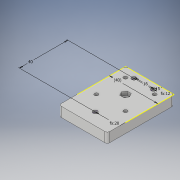
# Autodesk Inventor part: Laser_Mount
Saved by Autodesk Inventor 2019 (Build 230136000, 136)
## iProperties
Created: 2018-07-22
Part Number: Laser_Mount
Material: Generisch
Document SubType Name: Modeling
Designer: marc
Density: 1 g/cm^3
Appearance: Vorgabe
Author: marc
## iProperties of the stored document Laser_Mount_3D-Druck.ipt
Created: 2018-07-22
Part Number: Laser_Mount_3D-Druck
Material: Generisch
Document SubType Name: Modeling
Designer: marc
Density: 1 g/cm^3
Appearance: Vorgabe
Author: marc
Autodesk Inventor part; units mm, degrees
ref_plane "YZ Plane" through (0, 0, 0) normal (1, 0, 0) x (0, 1, 0)
ref_plane "XZ Plane" through (0, 0, 0) normal (0, 1, 0) x (-1, 0, 0)
ref_plane "XY Plane" through (0, 0, 0) normal (0, 0, 1) x (1, 0, 0)
sketch "Skizze1" plane through (0, 0, 0) normal (0, 1, 0) x (-1, 0, 0)
  line L0 (0, 0) -> (40, 0)
  line L1 (40, 0) -> (40, 40)
  line L2 (40, 40) -> (0, 40)
  line L3 (0, 40) -> (0, 0)
  dimension "d0" = 40
  dimension "d1" = 40
  constraints: 8 end point, 2 parallel, 1 horizontal, 1 perpendicular
  measures "d0" distance of L2.end L1.end
  measures "d1" distance of L1.end L0.end
extrude "Extrusion1" add sketch "Skizze1" along normal blind 8
sketch "Skizze2" plane through (0, 8, 0) normal (0, 1, 0) x (1, 0, 0)
  line L0 (-40, -40) -> (0, -40) projected
  line L1 (0, 0) -> (-40, 0) projected
  line L2 (0, -40) -> (0, 0) projected
  line L3 (-40, 0) -> (-40, -40) projected
  point P0 (-32, -32)
  point P1 (-32, -8)
  point P2 (-20, -20)
  point P3 (-8, -8)
  point P4 (-8, -32)
  dimension "d4" = 40
  dimension "d5" = 40
  dimension "d6" = 20
  dimension "d7" = 20
  dimension "d8" = 8
  dimension "d9" = 24
  dimension "d11" = 12
  dimension "d14" = 24
  constraints: 1 horizontal, 1 vertical alignment, 2 other
  measures "d4" distance between parallel lines of L0 L1
  measures "d5" distance between parallel lines of L2 L3
  measures "d6" distance from line of L1 point (-20, -20)
  measures "d7" distance from line of L2 point (-20, -20)
  measures "d8" distance from line of L1 point (-32, -8)
  measures "d9" distance of point (-32, -8) point (-32, -32)
  measures "d11" horizontal distance of point (-20, -20) point (-32, -32)
  measures "d14" distance of point (-32, -8) point (-8, -8)
hole "Bohrung1" at (-32, 8, 32) at (-32, 8, 8) at (-20, 8, 20) at (-8, 8, 8) at (-8, 8, 32) direction (0, -1, 0) diameter 3 end through all
sketch "Skizze3" plane through (0, 8, 0) normal (0, 1, 0) x (1, 0, 0)
  circle A0 centre (-20, -20) radius 1.5 projected
  line L0 (-21.7321, -17) -> (-18.2679, -17)
  line L1 (-18.2679, -17) -> (-16.5359, -20)
  line L2 (-16.5359, -20) -> (-18.2679, -23)
  line L3 (-18.2679, -23) -> (-21.7321, -23)
  line L4 (-21.7321, -23) -> (-23.4641, -20)
  line L5 (-23.4641, -20) -> (-21.7321, -17)
  line L6 (0, 0) -> (-40, 0) projected
  dimension "d26" = 6
  constraints: 12 end point, 1 coincident, 1 parallel, 13 other
  measures "d26" distance between parallel lines of L0 L3
extrude "Extrusion2" cut sketch "Skizze3" against normal blind 3
chamfer "Fase1" distance 0.5 angle 45 5 edges at (-32, 0, 6.5) (-32, 0, 30.5) (-8, 0, 30.5) (-8, 0, 6.5) (-20, 0, 18.5)
sketch "Skizze4" plane through (0, 8, 0) normal (0, 1, 0) x (1, 0, 0)
  line L0 (0, -40) -> (0, 0) projected
  line L1 (-40, 0) -> (-40, -40) projected
  line L2 (0, 0) -> (-40, 0) projected
  point P0 (-28, -5)
  point P1 (-12, -5)
  point P2 (-20, -45)
  dimension "d32" = 16
  dimension "d33" = 12
  dimension "d34" = 40
  dimension "d35" = 40
  dimension "d36" = 20
  dimension "d37" = 5
  constraints: 1 horizontal alignment
  measures "d32" distance of point (-12, -5) point (-28, -5)
  measures "d33" distance from line of L0 point (-12, -5)
  measures "d34" distance between parallel lines of L1 L0
  measures "d35" vertical distance of point (-20, -45) point (-12, -5)
  measures "d36" distance from line of L0 point (-20, -45)
  measures "d37" distance from line of L2 point (-12, -5)
move faces "Verschieben1" translate (0, 0, 15) faces at (-26.6667, 5.3333, 40)
sketch "Skizze5" plane through (0, 0, 0) normal (0, -1, 0) x (1, 0, 0)
  circle A0 centre (-8, 8) radius 2 projected
  circle A1 centre (-32, 32) radius 2 projected
  line L0 (0, 0) -> (-40, 0) projected
  line L1 (0, 55) -> (0, 0) projected
  line L2 (-40, 55) -> (0, 55) projected
  line L3 (-40, 0) -> (-40, 55) projected
  circle A2 centre (-32, 8) radius 2 projected
  circle A3 centre (-8, 32) radius 2 projected
  circle A4 centre (-20, 20) radius 2 projected
  point P0 (-12, 5)
  point P1 (-28, 5)
  point P2 (-20, 45)
hole "Bohrung2" at (-12, 0, 5) at (-28, 0, 5) at (-20, 0, 45) direction (0, 1, 0) diameter 3.6 end through all counterbore diameter 5.5 counterbore depth 3.2 clearance for "Sechskantkopfschraube ISO 24017" size "M3" standard "ISO"
fillet "Rundung1" radius 2 4 edges at (0, 4, 55) (-40, 4, 55) (0, 4, 0) (-40, 4, 0)
equation "\"d6\" = 0.5 * d4"
equation "\"d7\" = 0.5 * d5"
equation "\"d33\" = -0.5 * d32 + 0.5 * d34"
equation "\"d36\" = d33 + 0.5 * d32"
